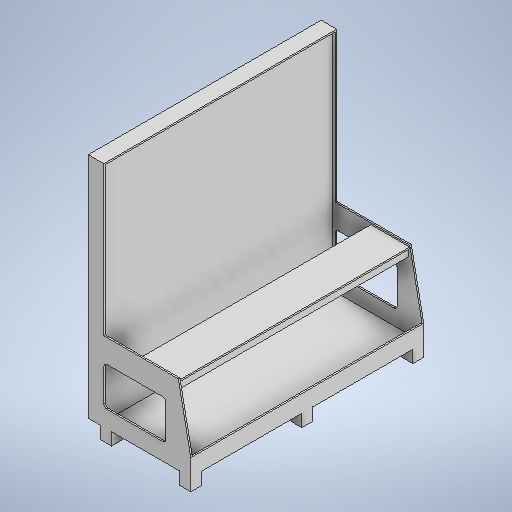
# Autodesk Inventor part: Стол приёма ГПХ
Saved by Autodesk Inventor 2025 (Build 290162010, 162A)
## iProperties
Created: 2025-12-01
Part Number: Стол приёма ГПХ
Material: Generic
Document SubType Name: Modeling
Designer: pokla
Density: 1 g/cm^3
Appearance: Default
Author: pokla
Autodesk Inventor part; units mm, degrees
ref_plane "YZ Plane" through (0, 0, 0) normal (1, 0, 0) x (0, 1, 0)
ref_plane "XZ Plane" through (0, 0, 0) normal (0, 1, 0) x (-1, 0, 0)
ref_plane "XY Plane" through (0, 0, 0) normal (0, 0, 1) x (1, 0, 0)
sketch "Sketch1" plane through (0, 0, 0) normal (0, 1, 0) x (-1, 0, 0)
  line L0 (0, 0) -> (0, 1550)
  line L1 (0, 1550) -> (-100, 1550)
  line L2 (-100, 1550) -> (-100, 590)
  line L3 (-100, 590) -> (-580, 590)
  line L4 (-580, 590) -> (-660, 190)
  line L5 (-660, 190) -> (-660, 0)
  line L6 (-660, 0) -> (0, 0)
  dimension "d0" = 1550
  dimension "d1" = 100
  dimension "d2" = 660
  dimension "d3" = 190
  dimension "d4" = 480
  dimension "d5" = 590
  constraints: 14 end point, 4 perpendicular, 1 parallel, 1 vertical
  measures "d0" distance of L0.start L0.end
  measures "d1" distance of L0.end L1.end
  measures "d2" distance of L5.end L0.start
  measures "d3" distance of L4.end L5.end
  measures "d4" distance of L2.end L3.end
  measures "d5" distance between parallel lines of L6 L3
extrude "Extrusion1" add sketch "Sketch1" along normal mid plane 1500
sketch "Sketch2" plane through (660, 750, 0) normal (0, 0, -1) x (-1, 0, 0)
  line L0 (0, -1500) -> (0, 0) projected
  line L1 (660, -1500) -> (0, -1500) projected
  line L2 (660, -1500) -> (660, 0) projected
  line L3 (0, 0) -> (660, 0) projected
  line L4 (0, -1500) -> (0, 0) projected
  line L5 (0, -1500) -> (70, -1500)
  line L6 (70, -1500) -> (70, -1430)
  line L7 (70, -1430) -> (0, -1430)
  line L8 (0, -1430) -> (0, -1500)
  line L9 (0, -785) -> (70, -785)
  line L10 (70, -785) -> (70, -715)
  line L11 (70, -715) -> (0, -715)
  line L12 (0, -715) -> (0, -785)
  line L13 (0, -70) -> (70, -70)
  line L14 (70, -70) -> (70, 0)
  line L15 (70, 0) -> (0, 0)
  line L16 (0, 0) -> (0, -70)
  line L17 (510, -1500) -> (580, -1500)
  line L18 (580, -1500) -> (580, -1430)
  line L19 (580, -1430) -> (510, -1430)
  line L20 (510, -1430) -> (510, -1500)
  line L21 (510, -785) -> (580, -785)
  line L22 (580, -785) -> (580, -715)
  line L23 (580, -715) -> (510, -715)
  line L24 (510, -715) -> (510, -785)
  line L25 (510, -70) -> (580, -70)
  line L26 (580, -70) -> (580, 0)
  line L27 (580, 0) -> (510, 0)
  line L28 (510, 0) -> (510, -70)
  point P0 (660, -750)
  point P1 (70, 0)
  point P2 (0, -715)
  point P3 (0, -1430)
  point P4 (70, -1500)
  dimension "d8" = 70
  dimension "d9" = 70
  dimension "d20" = 715
  dimension "d23" = 510
  constraints: 48 end point, 2 horizontal, 2 parallel, 1 perpendicular, 1 vertical, 40 other
  measures "d8" distance of L6.end L7.end
  measures "d9" distance of L5.end L6.end
  measures "d20" distance of L0.start L9.start
  measures "d23" distance of L0.start L17.start
extrude "Extrusion2" cut sketch "Sketch2" against normal blind 80 contours L0 L9 L10 L11 L13 L14 L3 L28 L25 L26 L2 L1 L18 L19 L20 L6 L7
sketch "Sketch3" plane through (0, -750, 1550) normal (-1, 0, 0) x (0, 0, 1)
  line L0 (0, 1500) -> (0, 0) projected
  line L1 (-1470, 1500) -> (0, 1500) projected
  line L2 (0, 0) -> (-1470, 0) projected
  line L3 (-1470, 1500) -> (-1470, 0) projected
  line L4 (-10, 1490) -> (-1460, 1490)
  line L5 (-1460, 1490) -> (-1460, 10)
  line L6 (-1460, 10) -> (-10, 10)
  line L7 (-10, 10) -> (-10, 1490)
  point P0 (-1550, 750)
  dimension "d28" = 10
  dimension "d30" = 10
  dimension "d31" = 10
  dimension "d32" = 10
  constraints: 8 end point, 2 parallel, 1 horizontal, 1 perpendicular
  measures "d28" distance between parallel lines of L0 L7
  measures "d30" distance between parallel lines of L1 L4
  measures "d31" distance between parallel lines of L2 L6
  measures "d32" distance between parallel lines of L3 L5
extrude "Extrusion3" cut sketch "Sketch3" against normal blind 70 contours L7 L6 L5 L4
sketch "Sketch4" plane through (0, -750, 0) normal (0, -1, 0) x (1, 0, 0)
  line L0 (120, 440) -> (480, 440)
  line L1 (500, 420) -> (500, 210)
  line L2 (480, 190) -> (120, 190)
  line L3 (100, 210) -> (100, 420)
  line L4 (0, 1550) -> (0, 80) projected
  line L5 (150, 80) -> (590, 80) projected
  arc A0 (120, 440) -> (100, 420) centre (120, 420) ccw
  arc A1 (100, 210) -> (120, 190) centre (120, 210) ccw
  arc A2 (480, 190) -> (500, 210) centre (480, 210) ccw
  arc A3 (500, 420) -> (480, 440) centre (480, 420) ccw
  point P0 (0, 0)
  point P1 (100, 440)
  point P2 (500, 190)
  point P3 (500, 440)
  dimension "d35" = 400
  dimension "d36" = 250
  dimension "d37" = 100
  dimension "d38" = 110
  dimension "d39" = 20
  constraints: 8 end point, 8 point on circle, 8 tangent, 6 point on line, 4 centre point, 3 equal radius, 2 parallel, 1 horizontal, 1 perpendicular
  measures "d35" distance of point (100, 440) point (500, 440)
  measures "d36" distance of point (500, 440) point (500, 190)
  measures "d37" distance between parallel lines of L4 L3
  measures "d38" distance between parallel lines of L5 L2
  measures "d39" radius of A0
extrude "Extrusion4" cut sketch "Sketch4" against normal through all
sketch "Sketch5" plane through (660, -750, 190) normal (1, 0, 0) x (0, 0, -1)
  line L0 (-1350, 10) -> (0, 10)
  line L1 (0, 10) -> (0, 1490)
  line L2 (0, 1490) -> (-1350, 1490)
  line L3 (-1350, 1490) -> (-1350, 10)
  line L4 (-1360, 1500) -> (-400, 1500) projected
  line L5 (-400, 0) -> (-1360, 0) projected
  line L6 (-1360, 0) -> (-1360, 1500) projected
  line L7 (0, 0) -> (0, 1500) projected
  point P0 (190, 750)
  point P1 (0, 750)
  point P2 (0, 750)
  dimension "d42" = 10
  dimension "d43" = 10
  dimension "d44" = 10
  constraints: 8 end point, 2 midpoint, 2 parallel, 1 coincident, 1 horizontal, 1 perpendicular
  measures "d42" distance between parallel lines of L4 L2
  measures "d43" distance between parallel lines of L5 L0
  measures "d44" distance between parallel lines of L6 L3
extrude "Extrusion5" cut sketch "Sketch5" against normal blind 580
sketch "Sketch6" plane through (120, -750, 190) normal (0, 0, 1) x (1, 0, 0)
  line L0 (-40, 1490) -> (530, 1490)
  line L1 (530, 1490) -> (530, 10)
  line L2 (530, 10) -> (-40, 10)
  line L3 (-40, 10) -> (-40, 1490)
  line L4 (540, 10) -> (540, 1490) projected
  line L5 (-20, 0) -> (-20, 1500) projected
  line L6 (-50, 10) -> (-50, 1490) projected
  point P0 (-120, 750)
  point P1 (245, 1490)
  point P2 (460, 1490)
  point P3 (245, 10)
  point P4 (460, 10)
  dimension "d47" = 10
  dimension "d50" = 10
  constraints: 8 end point, 2 horizontal alignment, 2 midpoint, 2 parallel, 1 horizontal, 1 perpendicular
  measures "d47" distance between parallel lines of L4 L1
  measures "d50" distance between parallel lines of L6 L3
extrude "Extrusion6" cut sketch "Sketch6" against normal blind 100
sketch "Sketch8" plane through (100, 740, 590) normal (0, -1, 0) x (1, 0, 0)
  line L0 (230, -10) -> (480, -10)
  line L1 (480, -10) -> (480, -20)
  line L2 (480, -20) -> (230, -20)
  line L3 (230, -20) -> (230, -10)
  line L4 (240, -20) -> (250, -20)
  line L5 (250, -20) -> (250, -70)
  line L6 (250, -70) -> (240, -70)
  line L7 (240, -70) -> (240, -20)
  line L8 (460, -20) -> (470, -20)
  line L9 (470, -20) -> (470, -70)
  line L10 (470, -70) -> (460, -70)
  line L11 (460, -70) -> (460, -20)
  line L12 (0, 0) -> (480, 0) projected
  point P0 (-100, -590)
  point P1 (480, -15)
  point P2 (470, -20)
  point P3 (250, -20)
  dimension "d51" = 250
  dimension "d52" = 10
  dimension "d53" = 10
  dimension "d54" = 10
  dimension "d55" = 10
  dimension "d56" = 10
  dimension "d57" = 50
  dimension "d58" = 10
  constraints: 24 end point, 6 parallel, 3 horizontal, 3 perpendicular, 3 point on line, 1 midpoint, 1 vertical alignment
  measures "d51" distance of L0.start L0.end
  measures "d52" distance between parallel lines of L2 L0
  measures "d53" distance between parallel lines of L7 L5
  measures "d54" distance between parallel lines of L11 L9
  measures "d55" distance between parallel lines of L3 L7
  measures "d56" distance between parallel lines of L9 L1
  measures "d57" distance of L4.end L5.end
  measures "d58" distance between parallel lines of L12 L0
extrude "Extrusion7" add sketch "Sketch8" along normal blind 1480
equation "\"d53\" = d52"
equation "\"d54\" = d52"
body "Solid1"
